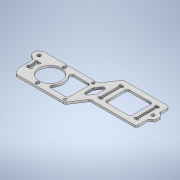
# Autodesk Inventor part: Ankle_side_frame
Saved by Autodesk Inventor 2020.4 (Build 244396000, 396)
## iProperties
Created: 2021-10-01
Part Number: Ankle_side_frame
Material: アルミニウム 2014-T4
Document SubType Name: Modeling
Designer: Masato Kubotera
Density: 2.8 g/cm^3
Appearance: 滑らか - 淡い灰色
Description: A2017 T2
Mass: 9.43206 g
Surface Area: 47.4383 cm^2
Volume: 3.36859 cm^3
Author: Masato Kubotera
Autodesk Inventor part; units mm, degrees
ref_plane "YZ Plane" through (0, 0, 0) normal (1, 0, 0) x (0, 1, 0)
ref_plane "XZ Plane" through (0, 0, 0) normal (0, 1, 0) x (-1, 0, 0)
ref_plane "XY Plane" through (0, 0, 0) normal (0, 0, 1) x (1, 0, 0)
sketch "スケッチ1" plane through (0, 0, 0) normal (0, 0, 1) x (1, 0, 0)
  line L0 (28, 13.5) -> (1, 13.5) construction
  line L1 (1, 13.5) -> (1, -13.5) construction
  line L2 (1, -13.5) -> (28, -13.5) construction
  line L3 (28, -13.5) -> (28, 13.5) construction
  line L4 (28, 13.5) -> (1, -13.5) construction
  line L5 (1, 13.5) -> (28, -13.5) construction
  circle A0 centre (0, 0) radius 10.5 construction
  circle A1 centre (0, 0) radius 10.75
  arc A2 (0, 16) -> (-12, 10.583) centre (0, 0) ccw construction
  line L6 (1, 0) -> (28, 0) construction
  line L7 (14.5, 13.5) -> (14.5, -13.5) construction
  circle A3 centre (28, 13.5) radius 1.35
  arc A4 (-0.35, 12.5) -> (2.35, 12.5) centre (1, 12.5) ccw
  line L8 (2.35, 13.5) -> (2.35, 12.5)
  line L9 (-0.35, 13.5) -> (-0.35, 12.5)
  arc A5 (2.35, 13.5) -> (-0.35, 13.5) centre (1, 13.5) ccw
  line L10 (-12, 10.583) -> (-12, -10.583) construction
  arc A6 (-12, -10.583) -> (0, -16) centre (0, 0) ccw construction
  circle A7 centre (28, -13.5) radius 1.35
  arc A8 (2.35, -12.5) -> (-0.35, -12.5) centre (1, -12.5) ccw
  line L11 (2.35, -13.5) -> (2.35, -12.5)
  line L12 (-0.35, -13.5) -> (-0.35, -12.5)
  arc A9 (-0.35, -13.5) -> (2.35, -13.5) centre (1, -13.5) ccw
  line L13 (-17.5, 5) -> (-14.5, 5) construction
  line L14 (-14.5, 5) -> (-14.5, -5) construction
  line L15 (-14.5, -5) -> (-17.5, -5) construction
  line L16 (-17.5, -5) -> (-17.5, 5) construction
  line L17 (-17.5, 5) -> (-14.5, -5) construction
  line L18 (-14.5, 5) -> (-17.5, -5) construction
  line L19 (-17.51, 5.01) -> (-14.49, 5.01)
  line L20 (-14.49, 5.01) -> (-14.49, 2.91) construction
  line L21 (-14.49, -5.01) -> (-17.51, -5.01)
  line L22 (-17.51, -5.01) -> (-17.51, -2.91) construction
  line L23 (-17.51, 5.01) -> (-14.49, -5.01) construction
  line L24 (-14.49, 5.01) -> (-17.51, -5.01) construction
  arc A10 (-17.51, 5.01) -> (-17.51, 2.91) centre (-17.51, 3.96) ccw
  line L25 (-17.5, 0) -> (-14.5, 0) construction
  line L26 (-16, 5) -> (-16, -5) construction
  arc A11 (-14.49, 2.91) -> (-14.49, 5.01) centre (-14.49, 3.96) ccw
  arc A12 (-17.51, -2.91) -> (-17.51, -5.01) centre (-17.51, -3.96) ccw
  arc A13 (-14.49, -5.01) -> (-14.49, -2.91) centre (-14.49, -3.96) ccw
  line L27 (-17.51, 2.91) -> (-17.51, 5.01) construction
  line L28 (-17.51, -2.91) -> (-17.51, 2.91)
  line L29 (-14.49, -2.91) -> (-14.49, -5.01) construction
  line L30 (-14.49, 2.91) -> (-14.49, -2.91)
  circle A14 centre (-21, 10.5) radius 1.55
  line L31 (-21, 7.0359) -> (-24, 8.7679) construction
  line L32 (-24, 8.7679) -> (-24, 12.2321) construction
  line L33 (-24, 12.2321) -> (-21, 13.9641) construction
  line L34 (-21, 13.9641) -> (-18, 12.2321) construction
  line L35 (-18, 12.2321) -> (-18, 8.7679) construction
  line L36 (-18, 8.7679) -> (-21, 7.0359) construction
  line L37 (-21.4737, 16) -> (-26, 13.3868)
  line L38 (-26, 13.3868) -> (-26, 7.6132)
  line L39 (-26, 7.6132) -> (-20.5, 4.4378)
  line L40 (-20.5, 4.4378) -> (-20.5, -10)
  line L41 (-20.5, -10) -> (-17.0359, -16)
  line L42 (-17.0359, -16) -> (30.4, -16)
  line L43 (-21.4737, 16) -> (30.4, 16)
  arc A15 (6.2732, -11.1) -> (6.2732, 11.1) centre (0, 0) ccw
  line L44 (6.2732, 11.1) -> (28, 11.1)
  circle A16 centre (28, 13.5) radius 2.4 construction
  circle A17 centre (28, -13.5) radius 2.4 construction
  line L45 (6.2732, -11.1) -> (28, -11.1)
  line L46 (79.5, 25.4) -> (77.5, 25.4) construction
  line L47 (77.5, 25.4) -> (77.5, 3.6) construction
  line L48 (77.5, 3.6) -> (79.5, 3.6) construction
  line L49 (79.5, 3.6) -> (79.5, 25.4) construction
  line L50 (79.5, 25.4) -> (77.5, 3.6) construction
  line L51 (77.5, 25.4) -> (79.5, 3.6) construction
  line L52 (77.49, 25.41) -> (79.51, 25.41)
  line L53 (79.51, 25.41) -> (79.51, 23.31) construction
  line L54 (79.51, 3.59) -> (77.49, 3.59)
  line L55 (77.49, 3.59) -> (77.49, 5.69) construction
  line L56 (77.49, 25.41) -> (79.51, 3.59) construction
  line L57 (79.51, 25.41) -> (77.49, 3.59) construction
  arc A18 (77.49, 25.41) -> (77.49, 23.31) centre (77.49, 24.36) ccw
  line L58 (78.5, 25.4) -> (78.5, 3.6) construction
  line L59 (77.5, 14.5) -> (79.5, 14.5) construction
  arc A19 (79.51, 23.31) -> (79.51, 25.41) centre (79.51, 24.36) ccw
  arc A20 (77.49, 5.69) -> (77.49, 3.59) centre (77.49, 4.64) ccw
  arc A21 (79.51, 3.59) -> (79.51, 5.69) centre (79.51, 4.64) ccw
  line L60 (77.49, 23.31) -> (77.49, 25.41) construction
  line L61 (79.51, 23.31) -> (79.51, 5.69)
  line L62 (79.51, 5.69) -> (79.51, 3.59) construction
  line L63 (77.49, 5.69) -> (77.49, 23.31)
  circle A22 centre (83.5, 15.5) radius 1.55
  line L64 (83.5, 12.0359) -> (80.5, 13.7679) construction
  line L65 (80.5, 13.7679) -> (80.5, 17.2321) construction
  line L66 (80.5, 17.2321) -> (83.5, 18.9641) construction
  line L67 (83.5, 18.9641) -> (86.5, 17.2321) construction
  line L68 (86.5, 17.2321) -> (86.5, 13.7679) construction
  line L69 (86.5, 13.7679) -> (83.5, 12.0359) construction
  line L70 (40, 30.4) -> (84.5, 30.4)
  line L71 (84.5, 30.4) -> (84.5, 20.6962)
  line L72 (84.5, 20.6962) -> (88.5, 18.3868)
  line L73 (88.5, 18.3868) -> (88.5, 12.6132)
  line L74 (88.5, 12.6132) -> (84.5, 10.3038)
  line L75 (84.5, 10.3038) -> (84.5, -1.4)
  line L76 (84.5, -1.4) -> (40, -1.4)
  line L77 (30.4, -16) -> (40, -1.4)
  line L78 (40, 30.4) -> (40, -1.4) construction
  line L79 (32, 9.3861) -> (32, -4.4659)
  line L80 (32, -4.4659) -> (39, 6.1799)
  line L81 (39, 6.1799) -> (39, 19.8861)
  line L82 (39, 19.8861) -> (32, 9.3861)
  line L83 (-17.5, 10) -> (-14.5, 10) construction
  line L84 (-15.0446, -6.3696) -> (-16.9554, -6.3696) construction
  line L85 (-17.5, 10) -> (-15.0446, -6.3696) construction
  line L86 (-14.5, 10) -> (-16.9554, -6.3696) construction
  line L87 (40, 30.4) -> (30.4, 16)
  line L88 (30.4, 16) -> (30.4, -16) construction
  line L89 (43, 25.5) -> (45, 25.5) construction
  line L90 (45, 25.5) -> (45, 3.5) construction
  line L91 (45, 3.5) -> (43, 3.5) construction
  line L92 (43, 3.5) -> (43, 25.5) construction
  line L93 (43, 25.5) -> (45, 3.5) construction
  line L94 (45, 25.5) -> (43, 3.5) construction
  line L95 (42.99, 25.51) -> (45.01, 25.51)
  line L96 (45.01, 25.51) -> (45.01, 23.41)
  line L97 (45.01, 3.49) -> (42.99, 3.49)
  line L98 (42.99, 3.49) -> (42.99, 5.59) construction
  line L99 (42.99, 25.51) -> (45.01, 3.49) construction
  line L100 (45.01, 25.51) -> (42.99, 3.49) construction
  line L101 (44, 25.5) -> (44, 3.5) construction
  line L102 (43, 14.5) -> (45, 14.5) construction
  arc A23 (42.99, 25.51) -> (42.99, 23.41) centre (42.99, 24.46) ccw
  arc A24 (45.01, 23.41) -> (45.01, 25.51) centre (45.01, 24.46) ccw
  arc A25 (42.99, 5.59) -> (42.99, 3.49) centre (42.99, 4.54) ccw
  arc A26 (45.01, 3.49) -> (45.01, 5.59) centre (45.01, 4.54) ccw
  line L103 (45.01, 23.41) -> (45.01, 5.59)
  line L104 (42.99, 5.59) -> (42.99, 25.51)
  line L105 (45.01, 5.59) -> (45.01, 3.49) construction
  line L106 (28, 11.1) -> (28, -11.1)
  line L107 (49, 25.4) -> (49, 3.6)
  line L108 (49, 3.6) -> (73.5, 3.6)
  line L109 (73.5, 3.6) -> (73.5, 25.4)
  line L110 (73.5, 25.4) -> (49, 25.4)
  point P0 (14.5, 0)
  point P1 (-16, 0)
  point P2 (-16, 0)
  point P3 (78.5, 14.5)
  point P4 (44, 14.5)
  dimension "d0" = 27
  dimension "d1" = 27
  dimension "d2" = 21
  dimension "d3" = 0.25
  dimension "d6" = 2.7
  dimension "d9" = 1
  dimension "d10" = 1.35
  dimension "d11" = 1
  dimension "d12" = 16
  dimension "d13" = 12
  dimension "d14" = 3
  dimension "d16" = 2.5
  dimension "d18" = 0.01
  dimension "d20" = 3.1
  dimension "d21" = 5.5
  dimension "d22" = 6
  dimension "d23" = 0.5
  dimension "d24" = 2
  dimension "d25" = 2
  dimension "d26" = 2
  dimension "d27" = 5
  dimension "d28" = 3
  dimension "d29" = 4.8
  dimension "d52" = 2
  dimension "d53" = 4.8
  dimension "d54" = 10
  dimension "d55" = 0.01
  dimension "d56" = 1.05
  dimension "d75" = 1.05
  dimension "d76" = 0.01
  dimension "d77" = 0.01
  dimension "d80" = 3.1
  dimension "d86" = 5
  dimension "d87" = 2
  dimension "d88" = 2
  dimension "d89" = 5
  dimension "d90" = 2
  dimension "d91" = 6
  dimension "d92" = 2
  dimension "d93" = 5
  dimension "d95" = 1
  dimension "d96" = 5
  dimension "d97" = 21.8
  dimension "d104" = 5
  dimension "d109" = 5
  dimension "d110" = 5
  dimension "d111" = 2
  dimension "d112" = 22
  dimension "d113" = 1.05
  dimension "d115" = 0.01
  dimension "d116" = 0.01
  dimension "d117" = 32.5
  dimension "d118" = 45
  dimension "d120" = 4
  dimension "d121" = 4
  dimension "d122" = 3
  dimension "d124" = 14.5
  dimension "d125" = 5
  dimension "d126" = 5
  dimension "d127" = 4
  dimension "d128" = 4
  constraints: 224 end point, 46 parallel, 38 point on circle, 33 midpoint, 28 symmetric about line, 27 centre point, 21 perpendicular, 16 point on line, 11 horizontal, 10 coincident, 7 tangent, 7 vertical, 3 collinear, 39 other
  measures "d0" distance of L2.end L1.end
  measures "d1" distance of L1.end L0.end
  measures "d2" diameter of A0
  measures "d3" radial gap between concentric circles of A1 A0
  measures "d6" diameter of A3
  measures "d9" distance of A4.centre L0.end
  measures "d10" radius of A5
  measures "d11" distance of point (0, 0) L6.start
  measures "d12" radius of A2
  measures "d13" distance from line of L10 A0.centre
  measures "d14" distance of L14.end L15.end
  measures "d16" distance between parallel lines of L10 L14
  measures "d18" distance between parallel lines of L19 L13
  measures "d20" diameter of A14
  measures "d21" distance from line of L13 A14.centre
  measures "d22" distance between parallel lines of L35 L32
  measures "d23" distance between parallel lines of L16 L35
  measures "d24" distance between parallel lines of L37 L33
  measures "d25" distance between parallel lines of L39 L31
  measures "d26" distance between parallel lines of L38 L32
  measures "d27" distance from line of L40.end L15
  measures "d28" distance between parallel lines of L40 L16
  measures "d29" diameter of A16
  measures "d52" radial gap between concentric circles of A1 A15
  measures "d53" diameter of A17
  measures "d54" distance between parallel lines of L15 L13
  measures "d55" distance between parallel lines of L16 L27
  measures "d56" radius of A10
  measures "d75" radius of A18
  measures "d76" distance between parallel lines of L46 L52
  measures "d77" distance between parallel lines of L55 L47
  measures "d80" diameter of A22
  measures "d86" distance between parallel lines of L71 L49
  measures "d87" distance between parallel lines of L73 L68
  measures "d88" distance between parallel lines of L72 L67
  measures "d89" horizontal distance of point (83.5, 15.5) point (78.5, 14.5)
  measures "d90" distance between parallel lines of L74 L69
  measures "d91" distance between parallel lines of L69 L66
  measures "d92" distance between parallel lines of L47 L49
  measures "d93" distance between parallel lines of L70 L46
  measures "d95" vertical distance of point (78.5, 14.5) A22.centre
  measures "d96" distance between parallel lines of L76 L48
  measures "d97" distance between parallel lines of L48 L46
  measures "d104" distance between parallel lines of L77 L80
  measures "d109" distance between parallel lines of L13 L83
  measures "d110" distance between parallel lines of L87 L82
  measures "d111" distance of L90.end L91.end
  measures "d112" distance of L89.end L90.end
  measures "d113" radius of A23
  measures "d115" distance between parallel lines of L95 L89
  measures "d116" distance between parallel lines of L98 L92
  measures "d117" distance between parallel lines of L47 L90
  measures "d118" distance from line of L90 point (0, 0)
  measures "d120" distance between parallel lines of L106 L79
  measures "d121" distance between parallel lines of L92 L81
  measures "d122" distance between parallel lines of L78 L92
  measures "d124" distance between parallel lines of L6 L102
  measures "d125" distance between parallel lines of L110 L70
  measures "d126" distance between parallel lines of L76 L108
  measures "d127" distance between parallel lines of L90 L107
  measures "d128" distance between parallel lines of L109 L47
extrude "押し出し1" add sketch "スケッチ1" along normal blind 2
fillet "フィレット1" radius 2 16 edges at (-21.4737, 16, 1) (-26, 13.3868, 1) (-26, 7.6132, 1) (-20.5, 4.4378, 1) (-20.5, -10, 1) (-17.0359, -16, 1) (30.4, 16, 1) (40, 30.4, 1) (84.5, 30.4, 1) (84.5, 20.6962, 1) (88.5, 18.3868, 1) (88.5, 12.6132, 1) (84.5, 10.3038, 1) (84.5, -1.4, 1) (40, -1.4, 1) (30.4, -16, 1)
fillet "フィレット2" radius 2 12 edges at (6.2732, 11.1, 1) (6.2732, -11.1, 1) (32, 9.3861, 1) (32, -4.4659, 1) (39, 6.1799, 1) (39, 19.8861, 1) (28, -11.1, 1) (28, 11.1, 1) (49, 25.4, 1) (49, 3.6, 1) (73.5, 3.6, 1) (73.5, 25.4, 1)
equation "\"d10\" = 0.5 * d6"
equation "\"d25\" = d24"
equation "\"d26\" = d24"
